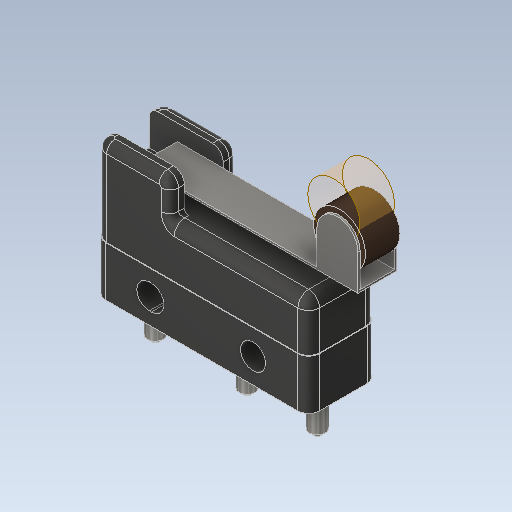
# Autodesk Inventor part: 49-0006
Saved by Autodesk Inventor 2021 (Build 250183000, 183)
## iProperties
Created: 2020-02-11
Part Number: 49-0006
Material: Generic
Document SubType Name: Modeling
Designer: Bradley
Density: 1 g/cm^3
Appearance: Smooth - Black
Author: Bradley
Autodesk Inventor part; units mm, degrees
ref_plane "YZ Plane" through (0, 0, 0) normal (1, 0, 0) x (0, 1, 0)
ref_plane "XZ Plane" through (0, 0, 0) normal (0, 1, 0) x (-1, 0, 0)
ref_plane "XY Plane" through (0, 0, 0) normal (0, 0, 1) x (1, 0, 0)
sketch "Sketch1" plane through (0, 0, 0) normal (0, 0, 1) x (1, 0, 0)
  line L0 (9.9, -2.3) -> (-9.9, -2.3)
  line L1 (-9.9, -2.3) -> (-9.9, 2.3)
  line L2 (-9.9, 2.3) -> (9.9, 2.3)
  line L3 (9.9, 2.3) -> (9.9, -2.3)
  line L4 (9.9, -2.3) -> (-9.9, 2.3) construction
  line L5 (-9.9, -2.3) -> (9.9, 2.3) construction
  circle A0 centre (4.75, 0) radius 1.15
  line L6 (-6, 0) -> (-3.5, 0) construction
  line L7 (-4.85, -1.15) -> (-4.65, -1.15)
  line L8 (-4.65, 1.15) -> (-4.85, 1.15)
  arc A1 (-4.85, 1.15) -> (-4.85, -1.15) centre (-4.85, 0) ccw
  arc A2 (-4.65, -1.15) -> (-4.65, 1.15) centre (-4.65, 0) ccw
  line L9 (4.75, 0) -> (-4.75, 0) construction
  line L10 (9.85, 2.3) -> (9.85, 6.9)
  line L11 (9.85, 6.9) -> (-9.85, 6.9)
  line L12 (-9.85, 6.9) -> (-9.85, 2.3)
  line L13 (-7.25, 8.7) -> (13.05, 8.7)
  line L14 (13.05, 8.7) -> (13.05, 8.5)
  line L15 (13.05, 8.5) -> (-7.25, 8.5)
  line L16 (-7.25, 8.5) -> (-7.25, 8.7)
  circle A3 centre (11.15, 11.8) radius 2.4
  line L17 (11.15, 11.8) -> (-7.25, 8.5) construction
  line L18 (-7.25, 8.5) -> (10.6284, 13.96) construction
  circle A4 centre (10.6284, 13.96) radius 2.4
  circle A5 centre (11.15, 11.8) radius 1.9 construction
  point P0 (0, 0)
  point P1 (0, 0)
  point P2 (0, 6.9)
  point P3 (0, 0)
  dimension "d0" = 19.8
  dimension "d1" = 4.6
  dimension "d2" = 2.3
  dimension "d3" = 2.5
  dimension "d4" = 9.5
  dimension "d7" = 19.7
  dimension "d8" = 6.9
  dimension "d11" = 6.4
  dimension "d12" = 11.8
  dimension "d13" = 4.8
  dimension "d14" = 8.7
  dimension "d15" = 0.2
  dimension "d16" = 12
  dimension "d21" = 2.16
  dimension "d24" = 3.8
  constraints: 40 end point, 7 midpoint, 6 centre point, 6 point on circle, 5 parallel, 5 tangent, 4 perpendicular, 4 point on line, 3 horizontal, 2 coincident, 2 equal radius, 1 collinear, 1 equal length, 1 vertical, 1 vertical alignment
  measures "d0" distance of L1.end L2.end
  measures "d1" distance of L0.end L1.end
  measures "d2" diameter of A0
  measures "d3" distance of L6.start L6.end
  measures "d4" distance of L9.start L9.end
  measures "d7" distance of L10.end L11.end
  measures "d8" distance from line of L9.start L11
  measures "d11" horizontal distance of L9.start L17.start
  measures "d12" vertical distance of L9.start L17.start
  measures "d13" diameter of A3
  measures "d14" distance from line of L9.start L13
  measures "d15" distance of L13.end L14.end
  measures "d16" distance from line of L9.start L16
  measures "d21" vertical distance of L17.start L18.end
  measures "d24" diameter of A5
extrude "Extrusion1" add sketch "Sketch1" along normal mid plane 6.4 contours L0 L1 L2 L3
extrude "Extrusion2" add sketch "Sketch1" along normal mid plane 6.3 contours L2 L12 L11 L10
extrude "Extrusion3" add sketch "Sketch1" along normal mid plane 3.6 contours L13 L14 L15 L16
extrude "Extrusion4" add sketch "Sketch1" along normal mid plane 3.2 contours A3 A4 | A4 A3 picked at (11.2706, 10.9018) picked at (10.8948, 12.4454)
surface extrude "ExtrusionSrf1" sketch "Sketch1" along normal mid plane 3.2 shown yes curves A4
sketch "Sketch2" plane through (0, 0, 1.8) normal (0, 0, 1) x (1, 0, 0)
  circle A0 centre (11.15, 11.8) radius 2.4 projected
  line L0 (13.05, 8.7) -> (-7.25, 8.7) projected
  line L1 (-7.25, 8.7) -> (-7.25, 8.5) projected
  line L2 (-7.25, 8.5) -> (13.05, 8.5) projected
  line L3 (13.05, 8.5) -> (13.05, 8.7) projected
  line L4 (13.05, 8.7) -> (13.05, 11.8)
  arc A1 (13.05, 11.8) -> (9.25, 11.8) centre (11.15, 11.8) ccw
  line L5 (9.25, 11.8) -> (9.25, 8.7)
  line L6 (9.85, 2.3) -> (9.85, 6.9) projected
  line L7 (9.85, 6.9) -> (-9.85, 6.9) projected
  line L8 (-9.85, 6.9) -> (-9.85, 2.3) projected
  line L9 (9.85, 2.3) -> (-9.85, 2.3) projected
  line L10 (-9.85, 6.9) -> (9.85, 6.9) projected
  line L11 (-9.85, 6.9) -> (-9.85, 10.2)
  line L12 (-9.85, 10.2) -> (-3, 10.2)
  line L13 (-3, 10.2) -> (-3, 6.9)
  point P0 (0, 0)
  dimension "d27" = 10.2
  dimension "d28" = 3
  constraints: 10 end point, 3 perpendicular, 2 point on circle, 2 point on line, 2 tangent, 2 vertical, 1 centre point, 1 concentric
  measures "d27" distance from line of point (0, 0) L12
  measures "d28" distance from line of point (0, 0) L13
extrude "Extrusion5" add sketch "Sketch2" against normal up to surface (0.2 mm away) contours L5 A1 L4 A0 | A0 L4 L0 L5 picked at (11.15, 11)
extrude "Extrusion6" add sketch "Sketch2" along normal up to surface (1.35 mm away) contours L13 L2 L1 L0 | L0 L1 L2 L13 L7 L11 L12
mirror "Mirror1" about plane through (0, 0, 0) normal (0, 0, 1) of "Extrusion6"
fillet "Fillet1" radius 1 13 edges at (-9.9, 0, 3.2) (-9.85, 6.25, 3.15) (3.425, 6.9, 3.15) (9.85, 6.9, 0) (9.85, 4.6, 3.15) (9.9, 0, 3.2) (9.85, 4.6, -3.15) (9.9, 0, -3.2) (-3, 10.2, 2.475) (-3, 10.2, -2.475) (-9.85, 6.25, -3.15) (3.425, 6.9, -3.15) (-9.9, 0, -3.2)
fillet "Fillet1" radius 0.8 6 edges at (-6.425, 10.2, -3.15) (-3, 8.55, -3.15) (-3, 8.55, 3.15) (-6.425, 10.2, 3.15) (-9.85, 10.2, -2.475) (-9.85, 10.2, 2.475)
fillet "Fillet1" radius 0.4 2 edges at (-3, 6.9, 2.475) (-3, 6.9, -2.475)
mirror "Mirror2" about plane through (0, 0, 0) normal (0, 0, 1) of "Extrusion5"
sketch "Sketch3" plane through (-8.9, -2.3, -3.2) normal (0, -1, 0) x (1, 0, 0)
  circle A0 centre (1.4, 3.2) radius 0.735
  circle A1 centre (9.9, 3.2) radius 0.735
  circle A2 centre (16.4, 3.2) radius 0.735
  line L0 (1.4, 3.2) -> (16.4, 3.2) construction
  point P0 (8.9, 3.2)
  point P1 (8.9, 3.2)
  dimension "d34" = 1.47
  dimension "d35" = 15
  dimension "d36" = 1
  constraints: 3 centre point, 2 end point, 2 equal radius, 1 coincident, 1 horizontal, 1 midpoint, 1 point on line
  measures "d34" diameter of A0
  measures "d35" distance of L0.start L0.end
  measures "d36" distance of point (8.9, 3.2) A1.centre
extrude "Extrusion7" add sketch "Sketch3" along normal blind 4.1
chamfer "Chamfer1" distance 0.4 angle 45 3 edges at (-8.235, -6.4, 0) (0.265, -6.4, 0) (6.765, -6.4, 0)
body "Solid1"
body "Srf1"
